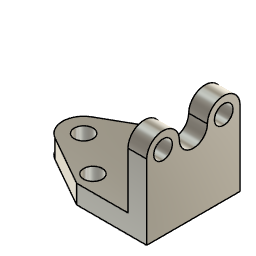
exercise04 (Autodesk Fusion 360 design; units mm, degrees)
Autodesk Fusion 360 part; units mm, degrees
sketch "草图1" plane through (0, 0, 0) normal (0, 0, 1) x (1, 0, 0)
  line L0 (0, -40) -> (0, 55) construction
  line L1 (-75, 0) -> (190, 0) construction
  line L2 (0, -35) -> (0, -32.2208) construction
  line L3 (0, -20) -> (0, 20)
  line L4 (0, 20) -> (-22, 20)
  line L5 (-22, 20) -> (-43.4432, 7.8267)
  line L6 (0, -20) -> (-22, -20)
  line L7 (-22, -20) -> (-43.4432, -7.8267)
  arc A0 (-43.4432, 7.8267) -> (-43.4432, -7.8267) centre (-39, 0) ccw
  circle A1 centre (-39, 0) radius 4
  circle A2 centre (-22, 13) radius 4
  circle A3 centre (-22, -13) radius 4
  dimension "d1" = 40
  dimension "d2" = 22
  dimension "d3" = 39
  dimension "d4" = 9
  dimension "d5" = 8
  dimension "d6" = 26
  dimension "d7" = 22
  constraint vertical L0
  constraint horizontal L1
  constraint coincident L0 L2.start
  constraint coincident L0 L2.end
  constraint coincident L0 L3.start
  constraint coincident L0 L3.end
  constraint perpendicular L3 L4
  constraint perpendicular L0 L6
  constraint symmetric L1 L3.start L3.end
  constraint symmetric L1 L5 L7
  constraint collinear origin L1.end A0.centre
  constraint equal L5 L7
  constraint tangent L5 A0
  constraint concentric A0 A1
  constraint symmetric L1 A2.centre A3.centre
  constraint equal A2 A3
  constraint equal A1 A2
  measures "d1" distance of L3.start L3.end
  measures "d2" distance of L3.end L4.end
  measures "d3" distance of L0 A0.centre
  measures "d4" radius of A0
  measures "d5" diameter of A1
  measures "d6" distance of A2.centre A3.centre
  measures "d7" distance of L3 A2.centre
extrude "拉伸1" add sketch "草图1" along normal blind 8
sketch "草图2" plane through (0, 0, 0) normal (1, 0, 0) x (0, 1, 0)
  line L0 (-20, 0) -> (20, 0)
  line L1 (20, 0) -> (20, 8)
  line L2 (20, 8) -> (-20, 8)
  line L3 (-20, 8) -> (-20, 0)
  line L4 (0, 39) -> (0, -13) construction
  line L5 (-35, 0) -> (42, 0) construction
  line L6 (-20, 0) -> (-20, 32)
  line L7 (20, 0) -> (20, 32)
  circle A0 centre (-13, 32) radius 4
  circle A1 centre (13, 32) radius 4
  arc A2 (-6, 32) -> (-20, 32) centre (-13, 32) ccw
  arc A3 (-6, 32) -> (6, 32) centre (0, 32) ccw
  arc A4 (20, 32) -> (6, 32) centre (13, 32) ccw
  dimension "d10" = 8
  dimension "d11" = 26
  dimension "d12" = 32
  constraint vertical L4
  constraint parallel L0 L5
  constraint coincident L0.start L3.end
  constraint perpendicular L5 L6
  constraint coincident L0.end L1.start
  constraint perpendicular L0 L7
  constraint tangent L6 A2
  constraint tangent L7 A4
  constraint equal L6 L7
  constraint equal A2 A4
  constraint equal A0 A1
  constraint concentric A1 A4
  constraint concentric A0 A2
  constraint collinear A0.centre A1.centre A3.centre
  constraint tangent A2 A3
  constraint tangent A3 A4
  measures "d10" diameter of A1
  measures "d11" distance of A0.centre A1.centre
  measures "d12" distance of L5 A1.centre
extrude "拉伸2" add sketch "草图2" along normal blind 8
sketch "草图3" plane through (0, 0, 0) normal (0, 1, 0) x (1, 0, 0)
  line L0 (0, -8) -> (-14, -8)
  line L1 (-14, -8) -> (0, -22)
  line L2 (0, -22) -> (0, -8)
  dimension "d15" = 14
  dimension "d16" = 14
  constraint horizontal L0
  constraint perpendicular L0 L2
  measures "d15" distance of L0.start L0.end
  measures "d16" distance of L0.start L1.end
extrude "拉伸3" add sketch "草图3" along normal mid plane 8
equation "d3 = 17 mm + 22 mm"
